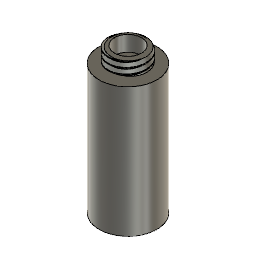
10) PLA Base Shaker Attachment (Autodesk Fusion 360 design; units mm, degrees)
Autodesk Fusion 360 part; units mm, degrees
ref_plane "WorkPlane1" through (0, 0, 0) normal (0, 0, 1) x (1, 0, 0)
sketch "Sketch1" plane through (0, 0, 0) normal (0, 0, 1) x (1, 0, 0)
  circle A0 centre (0, 0) radius 5.2
  circle A1 centre (0, 0) radius 7.5
  circle A2 centre (0, 0) radius 2.1
  dimension "d2" = 10.4
  dimension "d3" = 15
  dimension "d4" = 4.2
  constraint coincident A0.centre A1.centre
  measures "d2" diameter of A0
  measures "d3" diameter of A1
  measures "d4" diameter of A2
extrude "Extrude11" add sketch "Sketch1" along normal blind 32 contours A0 | A1 makes body 1
extrude "Extrude15" add 1 faces at (5.6643, -0.4769, 32) along direction (0, 0, 1) blind 4 separate body on bodies 1 makes body 2
extrude "Extrude16" add sketch "Sketch1" against normal blind 1.6 contours A1 bodies 1
sketch "Sketch11" plane through (0, 0, 36) normal (0, 0, 1) x (-1, 0, 0)
  circle A0 centre (0, 0) radius 2.1
  circle A1 centre (0, 0) radius 7.5
  circle A2 centre (0, 0) radius 3.5
  dimension "d67" = 7
  constraint coincident A0.centre A1.centre
  measures "d67" diameter of A2
extrude "Extrude17" cut sketch "Sketch11" against normal blind 4 contours A2 bodies 2
thread "Thread1" "ISO Metric profile 10.0 M10x1.5 M10x1.5 6g" major diameter 9.85 minor diameter 8.141 pitch 1.5 angle 60 modelled right hand crest width 0.2177 on face at (7.4627, -0.7468, 33.3333) crest through (4.925, 0, 31.625) on bodies 2
combine "Combine1" operation add target body 2 tool bodies 1
ref_plane "WorkPlane7" through (0, 0, 10) normal (0, 0, 1) x (1, 0, 0)
sketch "Sketch9" plane through (0, 0, 10) normal (0, 0, 1) x (1, 0, 0)
  circle A0 centre (0, 0) radius 3.9
  circle A1 centre (0, 0) radius 2.1
  dimension "d52" = 7.8
  measures "d52" diameter of A0
sketch "Sketch10" plane through (0, 0, 5) normal (0, 0, 1) x (-1, 0, 0)
  circle A0 centre (0, 0) radius 2.1
  circle A1 centre (0, 0) radius 7.5
loft "Loft1" [suppressed]
extrude "Extrude12" [suppressed]
extrude "Extrude13" [suppressed]
extrude "Extrude14" [suppressed]
fillet "Fillet2" [suppressed]
named bodies: "Bass Shaker 50mm M4 Bolt Adapter (Without sensor)", "Bass Shaker 50mm M4 Bolt Adapter Threaded"
